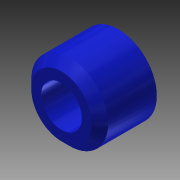
# Autodesk Inventor part: Roller
Saved by Autodesk Inventor 2015 (Build 190141000, 141)
## iProperties
Created: 2008-06-07
Part Number: Roller
Document SubType Name: Modeling
Designer: tangg
Density: 7.85 g/cm^3
Mass: 0.814587 g
Surface Area: 6.90277 cm^2
Volume: 0.814587 cm^3
Material: Non-Alloy Steel
Appearance: Blue - Wall Paint - Glossy
Author: tangg
Autodesk Inventor part; units mm, degrees
ref_plane "YZ Plane" through (0, 0, 0) normal (1, 0, 0) x (0, 1, 0)
ref_plane "XZ Plane" through (0, 0, 0) normal (0, 1, 0) x (-1, 0, 0)
sketch "Sketch1" plane through (0, 0, 0) normal (0, 0, 1) x (1, 0, 0)
  circle A0 centre (0, 0) radius 6
  circle A1 centre (0, 0) radius 3.175
  dimension "d4" = 6.35
  dimension "d5" = 12
  constraints: 2 centre point, 1 coincident
  measures "d4" diameter of A1
  measures "d5" diameter of A0
extrude "Extrusion2" add sketch "Sketch1" against normal blind 8.89
chamfer "Chamfer1" distance 1.27 angle 45 1 edges at (-6, 0, 0)
ref_plane "Work Plane1" through (0, 0, -2.54) normal (0, 0, 1) x (1, 0, 0)
body "Solid1"
